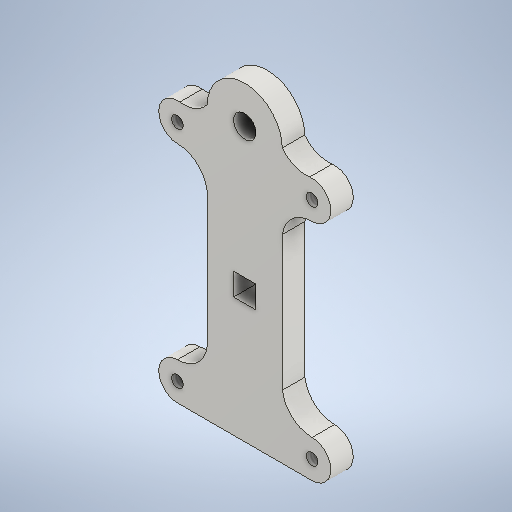
# Autodesk Inventor part: 23 - Valve Disc
Saved by Autodesk Inventor 2025.2 (Build 292293000, 293)
## iProperties
Created: 2025-07-29
Part Number: 23 - Valve Disc
Material: Steel AISI 1020 107 HR
Document SubType Name: Modeling
Designer: bless
Density: 7.87 g/cm^3
Appearance: Steel
Author: bless
Autodesk Inventor part; units mm, degrees
ref_plane "YZ Plane" through (0, 0, 0) normal (1, 0, 0) x (0, 1, 0)
ref_plane "XZ Plane" through (0, 0, 0) normal (0, 1, 0) x (-1, 0, 0)
ref_plane "XY Plane" through (0, 0, 0) normal (0, 0, 1) x (1, 0, 0)
sketch "Sketch1" plane through (0, 0, 0) normal (0, 0, 1) x (1, 0, 0)
  line L0 (-8.995, 0) -> (8.995, 0)
  arc A0 (8.995, 0) -> (8.995, 5) centre (8.995, 2.5) ccw
  arc A1 (-8.995, 5) -> (-8.995, 0) centre (-8.995, 2.5) ccw
  line L1 (-8.995, 0) -> (-8.995, 5) construction
  line L2 (8.995, 0) -> (8.995, 5) construction
  arc A2 (8.995, 30) -> (8.6755, 34.9795) centre (8.995, 32.5) ccw
  arc A3 (-8.6755, 34.9795) -> (-8.995, 30) centre (-8.995, 32.5) ccw
  line L3 (-1.5, 19) -> (1.5, 19)
  line L4 (1.5, 19) -> (1.5, 16)
  line L5 (1.5, 16) -> (-1.5, 16)
  line L6 (-1.5, 16) -> (-1.5, 19)
  line L7 (-1.5, 19) -> (1.5, 16) construction
  line L8 (1.5, 19) -> (-1.5, 16) construction
  line L9 (-8.995, 35.0339) -> (-8.995, 30) construction
  line L10 (8.995, 35.0339) -> (8.995, 30) construction
  line L11 (-5.0276, 26.51) -> (5.0276, 26.51) construction
  line L12 (5.0276, 26.51) -> (5.0276, 8.49)
  line L13 (5.0276, 8.49) -> (-5.0276, 8.49) construction
  line L14 (-5.0276, 8.49) -> (-5.0276, 26.51)
  line L15 (-5.0276, 26.51) -> (5.0276, 8.49) construction
  line L16 (5.0276, 26.51) -> (-5.0276, 8.49) construction
  arc A4 (8.995, 30) -> (5.0276, 26.51) centre (8.995, 26) ccw
  arc A5 (-5.0276, 26.51) -> (-8.995, 30) centre (-8.995, 26) ccw
  arc A6 (-8.995, 5) -> (-5.0276, 9.51) centre (-8.995, 9) ccw
  arc A7 (5.0276, 8.49) -> (8.995, 5) centre (8.995, 9) ccw
  arc A8 (5, 36.5) -> (-5, 36.5) centre (0, 36.5) ccw
  line L17 (-5, 36.5) -> (5, 36.5) construction
  arc A9 (-8.995, 35.0339) -> (-5, 36.5) centre (-8.1644, 38.9467) ccw
  arc A10 (5, 36.5) -> (8.995, 35.0339) centre (8.1644, 38.9467) ccw
  circle A11 centre (0, 36.5) radius 1.5
  point P0 (0, 0)
  point P1 (-8.995, 2.5)
  point P2 (8.995, 2.5)
  point P3 (0, 17.5)
  point P4 (-11.495, 32.5)
  point P5 (-11.495, 2.5)
  point P6 (0, 41.5)
  point P7 (11.495, 32.5)
  point P8 (11.495, 2.5)
  point P9 (-8.995, 32.5169)
  dimension "d1" = 2.5
  dimension "d2" = 2.5
  dimension "d3" = 2.5
  dimension "d4" = 32.5
  dimension "d6" = 3
  dimension "d7" = 3
  dimension "d8" = 16
  dimension "d12" = 18.02
  dimension "d13" = 4
  dimension "d14" = 4
  dimension "d16" = 5
  dimension "d17" = 4
  dimension "d22" = 41.5
  dimension "d25" = 22.99
  dimension "d29" = 3
  dimension "d30" = 36.5
  dimension "d33" = 8.995
  constraints: 36 end point, 30 point on circle, 12 centre point, 9 midpoint, 6 tangent, 5 equal radius, 5 parallel, 4 horizontal, 4 vertical alignment, 3 point on line, 2 perpendicular, 2 vertical, 1 coincident, 1 horizontal alignment
  measures "d1" radius of A0
  measures "d2" distance from line of L0 point (-8.995, 2.5)
  measures "d3" distance from line of L0 point (8.995, 2.5)
  measures "d4" distance from line of L0 A3.centre
  measures "d6" distance of L3.start L3.end
  measures "d7" distance of L3.end L4.end
  measures "d8" distance between parallel lines of L0 L5
  measures "d12" distance of L11.end L12.end
  measures "d13" radius of A5
  measures "d14" radius of A7
  measures "d16" radius of A8
  measures "d17" radius of A9
  measures "d22" distance from line of L0 point (0, 41.5)
  measures "d25" distance of point (11.495, 2.5) point (-11.495, 2.5)
  measures "d29" diameter of A11
  measures "d30" distance from line of L0 A8.centre
  measures "d33" horizontal distance of A8.centre A3.centre
extrude "Extrusion1" add sketch "Sketch1" along normal blind 3 contours A1 A6 L14 A5 A3 A9 A8 A10 A2 A4 L12 A7 A0 L0
sketch "Sketch2" plane through (0, 0, 3) normal (0, 0, 1) x (1, 0, 0)
  arc A0 (8.995, 30) -> (8.6755, 34.9795) centre (8.995, 32.5) ccw projected
  arc A1 (-8.6755, 34.9795) -> (-8.995, 30) centre (-8.995, 32.5) ccw projected
  arc A2 (-8.995, 5) -> (-8.995, 0) centre (-8.995, 2.5) ccw projected
  arc A3 (8.995, 0) -> (8.995, 5) centre (8.995, 2.5) ccw projected
  point P0 (0, 0)
  constraints: 4 coincident
hole "Hole1" at (-8.995, 32.5, 3) at (8.995, 32.5, 3) at (8.995, 2.5, 3) at (-8.995, 2.5, 3) direction (0, 0, -1) diameter 1.567 end through all thread size "M2x0.4" class "6H" standard "ANSI Metric M Profile"
body "Solid1"
